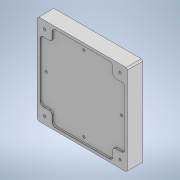
# Autodesk Inventor part: MDF_Block
Saved by Autodesk Inventor 2021 (Build 250183000, 183)
## iProperties
Created: 2020-07-24
Part Number: MDF_Block
Material: Generic
Document SubType Name: Modeling
Designer: CASE-SMALL2
Density: 1 g/cm^3
Appearance: Default
Author: CASE-SMALL2
Autodesk Inventor part; units mm, degrees
ref_plane "YZ Plane" through (0, 0, 0) normal (1, 0, 0) x (0, 1, 0)
ref_plane "XZ Plane" through (0, 0, 0) normal (0, 1, 0) x (-1, 0, 0)
ref_plane "XY Plane" through (0, 0, 0) normal (0, 0, 1) x (1, 0, 0)
sketch "Sketch1" plane through (0, 0, 0) normal (0, 0, 1) x (1, 0, 0)
  line L0 (-150, -150) -> (150, -150)
  line L1 (150, -150) -> (150, 150)
  line L2 (150, 150) -> (-150, 150)
  line L3 (-150, 150) -> (-150, -150)
  line L4 (-150, -150) -> (150, 150) construction
  line L5 (150, -150) -> (-150, 150) construction
  point P0 (0, 0)
  dimension "d0" = 300
  dimension "d1" = 300
  constraints: 12 end point, 2 midpoint, 2 parallel, 1 horizontal, 1 perpendicular
  measures "d0" distance of L2.end L0.start
  measures "d1" distance of L1.end L2.end
extrude "Extrusion1" add sketch "Sketch1" along normal blind 50
chamfer "Chamfer1" distance 5 angle 45 4 edges at (150, -150, 25) (150, 150, 25) (-150, 150, 25) (-150, -150, 25)
sketch "Sketch2" plane through (0, 0, 50) normal (0, 0, 1) x (1, 0, 0)
  line L0 (125, 194.8236) -> (125, -186.7434) construction
  line L1 (150, -145) -> (150, 145) construction
  line L2 (185.8456, 125) -> (-170.134, 125) construction
  line L3 (145, 150) -> (-145, 150) construction
  circle A0 centre (125, 125) radius 3.75
  circle A1 centre (125, 0) radius 3.75
  line L4 (-241.3299, 0) -> (257.0415, 0) construction
  line L5 (0, -263.0568) -> (0, 271.137) construction
  circle A2 centre (0, 125) radius 3.75
  circle A3 centre (125, -125) radius 3.75
  circle A4 centre (0, -125) radius 3.75
  line L6 (-150, -145) -> (-150, 145) construction
  circle A5 centre (-125, 125) radius 3.75
  circle A6 centre (-125, 0) radius 3.75
  circle A7 centre (-125, -125) radius 3.75
  point P0 (0, 0)
  point P1 (145, -150)
  point P2 (-125, 194.8236)
  point P3 (-185.8456, 125)
  point P4 (-145, -150)
  dimension "d7" = 25
  dimension "d8" = 125
  dimension "d9" = 25
  dimension "d10" = 7.5
  dimension "d11" = 7.5
  dimension "d12" = 7.5
  constraints: 11 symmetric about line, 8 centre point, 6 end point, 6 point on line, 1 horizontal, 1 vertical, 5 other
  measures "d7" distance between parallel lines of L1 L0
  measures "d8" distance from line of point (0, 0) L0
  measures "d9" distance between parallel lines of L3 L2
  measures "d10" diameter of A1
  measures "d11" diameter of A2
  measures "d12" diameter of A0
extrude "Extrusion2" cut sketch "Sketch2" against normal through all
sketch "Sketch3" plane through (0, 0, 50) normal (0, 0, 1) x (1, 0, 0)
  line L0 (-100, 140) -> (100, 140)
  line L1 (100, 140) -> (100, -140)
  line L2 (100, -140) -> (-100, -140)
  line L3 (-100, -140) -> (-100, 140)
  line L4 (-100, 140) -> (100, -140) construction
  line L5 (100, 140) -> (-100, -140) construction
  line L6 (-140, 100) -> (140, 100)
  line L7 (140, 100) -> (140, -100)
  line L8 (140, -100) -> (-140, -100)
  line L9 (-140, -100) -> (-140, 100)
  line L10 (-140, 100) -> (140, -100) construction
  line L11 (140, 100) -> (-140, -100) construction
  line L12 (150, -145) -> (150, 145) projected
  line L13 (145, 150) -> (-145, 150) projected
  line L14 (-145, -150) -> (145, -150) projected
  point P0 (0, 0)
  point P1 (100, 100)
  point P2 (-100, 100)
  point P3 (-100, -100)
  point P4 (100, -100)
  dimension "d15" = 10
  dimension "d16" = 10
  dimension "d17" = 50
  dimension "d18" = 50
  constraints: 24 end point, 4 midpoint, 4 parallel, 2 horizontal, 2 perpendicular
  measures "d15" distance between parallel lines of L12 L7
  measures "d16" distance between parallel lines of L13 L0
  measures "d17" distance between parallel lines of L12 L1
  measures "d18" distance between parallel lines of L14 L8
extrude "Extrusion3" cut sketch "Sketch3" against normal blind 5
fillet "Fillet1" radius 10 12 edges at (-100, 100, 47.5) (-100, -100, 47.5) (100, -100, 47.5) (100, 100, 47.5) (140, 100, 47.5) (140, -100, 47.5) (100, -140, 47.5) (-100, -140, 47.5) (-140, -100, 47.5) (-140, 100, 47.5) (-100, 140, 47.5) (100, 140, 47.5)
chamfer "Chamfer2" distance 1 angle 45 24 edges at (100, 120, 50) (102.9289, 102.9289, 50) (120, 100, 50) (137.0711, 97.0711, 50) (140, 0, 50) (137.0711, -97.0711, 50) (120, -100, 50) (102.9289, -102.9289, 50) (100, -120, 50) (97.0711, -137.0711, 50) (0, -140, 50) (-97.0711, -137.0711, 50) (-100, -120, 50) (-102.9289, -102.9289, 50) (-120, -100, 50) (-137.0711, -97.0711, 50) (-140, 0, 50) (-137.0711, 97.0711, 50) (-120, 100, 50) (-102.9289, 102.9289, 50) (-100, 120, 50) (-97.0711, 137.0711, 50) (0, 140, 50) (97.0711, 137.0711, 50)
equation "\"d1\" = d0"
equation "\"d9\" = d7"
equation "\"d11\" = d10"
equation "\"d12\" = d10"
equation "\"d18\" = d17"
body "Solid1"
